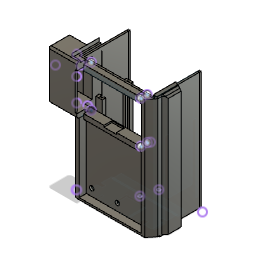
BAL-BOT-W-DISPLAY (Autodesk Fusion 360 design; units mm, degrees)
Autodesk Fusion 360 part; units mm, degrees
note: some values were not read from the file. Set by a fixed rule: which face or edge a step refers to.
(part 1 of 4)
sketch "Sketch1" plane through (0, 0, 0) normal (0, 1, 0) x (1, 0, 0)
  line L0 (0, 0) -> (-315, 0)
  line L1 (-315, 0) -> (-315, 66)
  line L2 (-315, 66) -> (0, 66)
  line L3 (0, 66) -> (0, 0)
  line L4 (-315, 0) -> (-272.5, 0)
  line L5 (-272.5, 0) -> (-272.5, -56.2)
  line L6 (-272.5, -56.2) -> (-315, -56.2)
  line L7 (-315, -56.2) -> (-315, 0)
  line L8 (0, 0) -> (-42.5, 0)
  line L9 (-42.5, 0) -> (-42.5, -56.2)
  line L10 (-42.5, -56.2) -> (0, -56.2)
  line L11 (0, -56.2) -> (0, 0)
  line L12 (-272.5, -56.2) -> (-42.5, -56.2)
  line L13 (-42.5, -56.2) -> (-42.5, 0)
  line L14 (-42.5, 0) -> (-272.5, 0)
  line L15 (-272.5, 0) -> (-272.5, -56.2)
  line L16 (-315, 0) -> (-272.5, -56.2)
  line L17 (0, 0) -> (-42.5, -56.2)
  dimension "d1" = 315
  dimension "d2" = 66
  dimension "d3" = 42.5
  dimension "d4" = 56.2
  dimension "d5" = 42.5
  dimension "d6" = 56.2
  constraint horizontal L0
  constraint vertical L1
  constraint horizontal L2
  constraint vertical L3
  constraint coincident L0.start L3.end
  constraint horizontal L4
  constraint vertical L5
  constraint horizontal L6
  constraint vertical L7
  constraint horizontal L8
  constraint vertical L9
  constraint horizontal L10
  constraint vertical L11
  constraint horizontal L12
  constraint vertical L13
  constraint horizontal L14
  constraint vertical L15
  measures "d1" distance of L0.start L0.end
  measures "d2" distance of L0.start L2.end
  measures "d3" distance of L0.end L4.end
  measures "d4" distance of L0.end L6.end
  measures "d5" distance of L0.start L8.end
  measures "d6" distance of L0.start L10.end
extrude "Extrude1" add sketch "Sketch1" along normal blind 5 contours L0 L8 L9 L13 L17 | L0 L1 L2 L3 L4 L8 L14 | L0 L5 L9 L12 L13 L14 L15 | L0 L4 L5 L15 L16 makes body 1
sketch "Sketch2" plane through (0, 5, 0) normal (0, 1, 0) x (-1, 0, 0)
  line L0 (315, 0) -> (272.5, 56.2)
  line L1 (272.5, 56.2) -> (42.5, 56.2)
  line L2 (42.5, 56.2) -> (0, 0)
  line L3 (0, 0) -> (0, -66)
  line L4 (0, -66) -> (315, -66)
  line L5 (315, -66) -> (315, 0)
  line L6 (272.5, 56.2) -> (272.5, -66)
  line L7 (42.5, 56.2) -> (42.5, -66)
  constraint coincident L0.end L1.start
  constraint coincident L4 L6.end
  constraint perpendicular L4 L6
  constraint coincident L1.end L2.start
  constraint coincident L4 L7.end
  constraint perpendicular L4 L7
extrude "Extrude2" cut sketch "Sketch2" against normal blind 5 contours L0 L4 L5 L6 | L2 L3 L4 L7 bodies 1
sketch "Sketch3" plane through (0, 5, 0) normal (0, 1, 0) x (-1, 0, 0)
  line L0 (272.5, -66) -> (272.5, 56.2)
  line L1 (272.5, 56.2) -> (42.5, 56.2)
  line L2 (42.5, 56.2) -> (42.5, -66)
  line L3 (42.5, -66) -> (272.5, -66)
  line L4 (42.5, -66) -> (152, -66)
  line L5 (152, -66) -> (152, -53.875)
  line L6 (152, -53.875) -> (42.5, -53.875)
  line L7 (42.5, -53.875) -> (42.5, -66)
  circle A0 centre (152, -53.875) radius 4
  line L8 (272.5, -66) -> (163, -66)
  line L9 (163, -66) -> (163, -12.125)
  line L10 (163, -12.125) -> (272.5, -12.125)
  line L11 (272.5, -12.125) -> (272.5, -66)
  circle A1 centre (163, -12.125) radius 4
  line L12 (272.5, -66) -> (259, -66)
  line L13 (259, -66) -> (259, -46)
  line L14 (259, -46) -> (272.5, -46)
  line L15 (272.5, -46) -> (272.5, -66)
  line L16 (259, -46) -> (56, -46)
  line L17 (56, -46) -> (56, -20)
  line L18 (56, -20) -> (259, -20)
  line L19 (259, -20) -> (259, -46)
  dimension "d11" = 109.5
  dimension "d12" = 12.125
  dimension "d13" = 8
  dimension "d14" = 109.5
  dimension "d15" = 53.875
  dimension "d16" = 8
  dimension "d17" = 13.5
  dimension "d18" = 20
  dimension "d19" = 203
  dimension "d20" = 26
  constraint horizontal L4
  constraint vertical L5
  constraint horizontal L6
  constraint vertical L7
  constraint coincident L2.end L3.start
  constraint coincident L5.end L6.start
  constraint horizontal L8
  constraint vertical L9
  constraint horizontal L10
  constraint vertical L11
  constraint coincident L0.start L3.end
  constraint coincident L9.end L10.start
  constraint horizontal L12
  constraint vertical L13
  constraint horizontal L14
  constraint vertical L15
  constraint horizontal L16
  constraint vertical L17
  constraint horizontal L18
  constraint vertical L19
  measures "d11" distance of L2.end L4.end
  measures "d12" distance of L2.end L6.end
  measures "d13" diameter of A0
  measures "d14" distance of L0.start L8.end
  measures "d15" distance of L0.start L10.end
  measures "d16" diameter of A1
  measures "d17" distance of L0.start L12.end
  measures "d18" distance of L0.start L14.end
  measures "d19" distance of L13.end L16.end
  measures "d20" distance of L13.end L18.end
extrude "Extrude3" cut sketch "Sketch3" against normal blind 5 contours L9 L16 L18 L19 | L9 L10 A1 | L9 L10 A1 | L9 L16 L17 L18 | L5 L6 A0 | L5 L6 A0 bodies 1
sketch "Sketch4" plane through (0, 0, 0) normal (0, -1, 0) x (1, 0, 0)
  line L0 (-56, -20) -> (-56, -46)
  line L1 (-56, -46) -> (-259, -46)
  line L2 (-259, -46) -> (-259, -20)
  line L3 (-259, -20) -> (-56, -20)
  circle A0 centre (-152, -53.875) radius 4
  circle A1 centre (-163, -12.125) radius 4
  line L4 (-272.5, 56.2) -> (-272.5, -66)
  line L5 (-272.5, -66) -> (-42.5, -66)
  line L6 (-42.5, -66) -> (-42.5, 56.2)
  line L7 (-42.5, 56.2) -> (-272.5, 56.2)
  line L8 (-42.5, 56.2) -> (-272.5, 56.2)
  line L9 (-272.5, 56.2) -> (-272.5, 51.2)
  line L10 (-272.5, 51.2) -> (-42.5, 51.2)
  line L11 (-42.5, 51.2) -> (-42.5, 56.2)
  line L12 (-42.5, 51.2) -> (-45, 51.2)
  line L13 (-45, 51.2) -> (-45, 3)
  line L14 (-45, 3) -> (-42.5, 3)
  line L15 (-42.5, 3) -> (-42.5, 51.2)
  line L16 (-272.5, 51.2) -> (-270, 51.2)
  line L17 (-270, 51.2) -> (-270, 3)
  line L18 (-270, 3) -> (-272.5, 3)
  line L19 (-272.5, 3) -> (-272.5, 51.2)
  line L20 (-45, 3) -> (-270, 3)
  line L21 (-270, 3) -> (-270, 51.2)
  line L22 (-270, 51.2) -> (-45, 51.2)
  line L23 (-45, 51.2) -> (-45, 3)
  dimension "d23" = 5
  dimension "d24" = 2.5
  dimension "d25" = 48.2
  dimension "d26" = 2.5
  dimension "d27" = 48.2
  constraint horizontal L8
  constraint vertical L9
  constraint horizontal L10
  constraint vertical L11
  constraint coincident L6.end L7.start
  constraint horizontal L12
  constraint vertical L13
  constraint horizontal L14
  constraint vertical L15
  constraint horizontal L16
  constraint vertical L17
  constraint horizontal L18
  constraint vertical L19
  constraint horizontal L20
  constraint vertical L21
  constraint horizontal L22
  constraint vertical L23
  measures "d23" distance of L6.end L10.end
  measures "d24" distance of L10.end L12.end
  measures "d25" distance of L10.end L14.end
  measures "d26" distance of L9.end L16.end
  measures "d27" distance of L9.end L18.end
extrude "Extrude4" cut sketch "Sketch4" against normal blind 5 contours L10 L13 L17 L20 L21 L22 L23 bodies 1
extrude "Extrude5" add 1 faces at (-270, 1.6667, 35.1333) along direction (1, 0, 0) blind 85 on bodies 1 bodies 1
extrude "Extrude6" add 1 faces at (-45, 1.6667, 35.1333) along direction (-1, 0, 0) blind 85 on bodies 1 bodies 1
sketch "Sketch5" plane through (0, 5, 0) normal (0, 1, 0) x (-1, 0, 0)
  line L0 (185, 3) -> (130, 3)
  line L1 (130, 3) -> (130, 51.2)
  line L2 (130, 51.2) -> (185, 51.2)
  line L3 (185, 51.2) -> (185, 3)
  line L4 (56, -46) -> (56, -20)
  line L5 (56, -20) -> (259, -20)
  line L6 (259, -20) -> (259, -46)
  line L7 (259, -46) -> (56, -46)
  circle A0 centre (152, -53.875) radius 4
  circle A1 centre (163, -12.125) radius 4
  line L8 (272.5, -66) -> (272.5, 56.2)
  line L9 (272.5, 56.2) -> (42.5, 56.2)
  line L10 (42.5, 56.2) -> (42.5, -66)
  line L11 (42.5, -66) -> (272.5, -66)
  line L12 (272.5, 56.2) -> (42.5, 56.2)
  line L13 (42.5, 56.2) -> (42.5, 51.2)
  line L14 (42.5, 51.2) -> (272.5, 51.2)
  line L15 (272.5, 51.2) -> (272.5, 56.2)
  dimension "d34" = 5
  constraint horizontal L12
  constraint vertical L13
  constraint horizontal L14
  constraint vertical L15
  constraint coincident L10 L13.end
  constraint coincident L8.end L9.start
  measures "d34" distance of L8.end L14.end
extrude "Extrude7" add sketch "Sketch5" along normal blind 150 contours L2 L8 L9 L10 L12 L13 L14 L15 bodies 1
sketch "Sketch6" plane through (0, 5, 0) normal (0, 1, 0) x (-1, 0, 0)
  line L0 (130, 51.2) -> (42.5, 51.2)
  line L1 (42.5, 51.2) -> (42.5, -66)
  line L2 (42.5, -66) -> (272.5, -66)
  line L3 (272.5, -66) -> (272.5, 51.2)
  line L4 (272.5, 51.2) -> (185, 51.2)
  line L5 (185, 51.2) -> (185, 3)
  line L6 (185, 3) -> (130, 3)
  line L7 (130, 3) -> (130, 51.2)
  line L8 (56, -46) -> (56, -20)
  line L9 (56, -20) -> (259, -20)
  line L10 (259, -20) -> (259, -46)
  line L11 (259, -46) -> (56, -46)
  circle A0 centre (152, -53.875) radius 4
  circle A1 centre (163, -12.125) radius 4
  line L12 (56, -20) -> (66, -20)
  line L13 (66, -20) -> (66, 51.2)
  line L14 (66, 51.2) -> (56, 51.2)
  line L15 (56, 51.2) -> (56, -20)
  line L16 (259, -20) -> (249, -20)
  line L17 (249, -20) -> (249, 51.2)
  line L18 (249, 51.2) -> (259, 51.2)
  line L19 (259, 51.2) -> (259, -20)
  point P0 (259, -20)
  dimension "d37" = 10
  dimension "d38" = 10
  dimension "d39" = 71.2
  constraint horizontal L12
  constraint vertical L13
  constraint horizontal L14
  constraint vertical L15
  constraint coincident L0 L13.end
  constraint coincident L8.end L9.start
  constraint horizontal L16
  constraint vertical L17
  constraint horizontal L18
  constraint vertical L19
  constraint coincident P0 L9.end
  measures "d37" distance of L8.end L12.end
  measures "d38" distance of P0 L16.end
  measures "d39" distance of P0 L18.end
extrude "Extrude8" add sketch "Sketch6" along normal blind 150 contours L0 L9 L12 L13 L14 L15 | L4 L9 L16 L17 L18 L19 bodies 1
sketch "Sketch7" plane through (-42.5, 0, 0) normal (1, 0, 0) x (0, 0, -1)
  line L0 (-56.2, 155) -> (-56.2, 0)
  line L1 (-56.2, 0) -> (66, 0)
  line L2 (66, 0) -> (66, 5)
  line L3 (66, 5) -> (-51.2, 5)
  line L4 (-51.2, 5) -> (-51.2, 155)
  line L5 (-51.2, 155) -> (-56.2, 155)
  line L6 (-51.2, 5) -> (-56.2, 5)
  line L7 (-56.2, 5) -> (-56.2, 155)
  line L8 (-56.2, 155) -> (-51.2, 155)
  line L9 (-51.2, 155) -> (-51.2, 5)
  constraint horizontal L6
  constraint vertical L7
  constraint horizontal L8
  constraint vertical L9
  constraint coincident L0.start L5.end
  constraint coincident L3.end L4.start
extrude "Extrude9" cut sketch "Sketch7" against normal blind 13.5 contours L0 L4 L5 L6 L7 L8 L9 bodies 1
sketch "Sketch8" plane through (-272.5, 0, 0) normal (-1, 0, 0) x (0, 0, 1)
  line L0 (51.2, 5) -> (-66, 5)
  line L1 (-66, 5) -> (-66, 0)
  line L2 (-66, 0) -> (56.2, 0)
  line L3 (56.2, 0) -> (56.2, 155)
  line L4 (56.2, 155) -> (51.2, 155)
  line L5 (51.2, 155) -> (51.2, 5)
  line L6 (51.2, 5) -> (56.2, 5)
  line L7 (56.2, 5) -> (56.2, 155)
  line L8 (56.2, 155) -> (51.2, 155)
  line L9 (51.2, 155) -> (51.2, 5)
  constraint horizontal L6
  constraint vertical L7
  constraint horizontal L8
  constraint vertical L9
  constraint coincident L3.end L4.start
  constraint coincident L0.start L5.end
extrude "Extrude10" cut sketch "Sketch8" against normal blind 13.5 contours L3 L4 L5 L6 L7 L8 L9 bodies 1
sketch "Sketch9" plane through (0, 0, -20) normal (0, 0, -1) x (-1, 0, 0)
  line L0 (56, 5) -> (56, 0)
  line L1 (56, 0) -> (259, 0)
  line L2 (259, 0) -> (259, 5)
  line L3 (259, 5) -> (259, 155)
  line L4 (259, 155) -> (249, 155)
  line L5 (249, 155) -> (249, 5)
  line L6 (249, 5) -> (66, 5)
  line L7 (66, 5) -> (66, 155)
  line L8 (66, 155) -> (56, 155)
  line L9 (56, 155) -> (56, 5)
  line L10 (56, 155) -> (66, 155)
  line L11 (66, 155) -> (66, 0)
  line L12 (66, 0) -> (56, 0)
  line L13 (56, 0) -> (56, 155)
  line L14 (249, 155) -> (259, 155)
  line L15 (259, 155) -> (259, 0)
  line L16 (259, 0) -> (249, 0)
  line L17 (249, 0) -> (249, 155)
  constraint horizontal L10
  constraint vertical L11
  constraint horizontal L12
  constraint vertical L13
  constraint coincident L1 L11.end
  constraint coincident L8.end L9.start
  constraint horizontal L14
  constraint vertical L15
  constraint horizontal L16
  constraint vertical L17
  constraint coincident L1.end L2.start
  constraint coincident L4.end L5.start
extrude "Extrude11" add sketch "Sketch9" along normal blind 25 contours L0 L1 L7 L8 L9 L10 L11 L12 L13 | L1 L2 L3 L4 L5 L14 L15 L16 L17 bodies 1
extrude "Extrude12" add 1 faces at (-62.6667, 53.3333, -45) along direction (0, 0, -1) blind 1 on bodies 1 bodies 1
extrude "Extrude13" add 1 faces at (-252.3333, 53.3333, -45) along direction (0, 0, -1) blind 1 on bodies 1 bodies 1
sketch "Sketch10" plane through (0, 0, 0) normal (0, -1, 0) x (1, 0, 0)
  line L0 (-185, 51.2) -> (-130, 51.2)
  line L1 (-130, 51.2) -> (-130, 3)
  line L2 (-130, 3) -> (-185, 3)
  line L3 (-185, 3) -> (-185, 51.2)
  line L4 (-66, -20) -> (-66, -46)
  line L5 (-66, -46) -> (-249, -46)
  line L6 (-249, -46) -> (-249, -20)
  line L7 (-249, -20) -> (-66, -20)
  circle A0 centre (-152, -53.875) radius 4
  circle A1 centre (-163, -12.125) radius 4
  line L8 (-42.5, -66) -> (-42.5, 56.2)
  line L9 (-42.5, 56.2) -> (-272.5, 56.2)
extrude "Extrude14" add 1 faces at (-62.6667, 105, -46) along direction (0, 0, -1) blind 20 on bodies 1 bodies 1
extrude "Extrude15" add 1 faces at (-252.3333, 55, -46) along direction (0, 0, -1) blind 20 on bodies 1 bodies 1
sketch "Sketch11" plane through (0, 5, 0) normal (0, 1, 0) x (-1, 0, 0)
  line L0 (249, -66) -> (249, -46)
  line L1 (249, -46) -> (66, -46)
  line L2 (66, -46) -> (66, -66)
  line L3 (66, -66) -> (249, -66)
  circle A0 centre (152, -53.875) radius 4
  line L4 (66, -66) -> (249, -66)
  line L5 (249, -66) -> (249, -61)
  line L6 (249, -61) -> (66, -61)
  line L7 (66, -61) -> (66, -66)
  dimension "d56" = 5
  constraint horizontal L4
  constraint vertical L5
  constraint horizontal L6
  constraint vertical L7
  constraint coincident L2.end L3.start
  measures "d56" distance of L2.end L6.end
extrude "Extrude16" add sketch "Sketch11" along normal blind 30 contours L0 L2 L3 L4 L5 L6 L7 bodies 1
sketch "Sketch12" plane through (0, 0, -66) normal (0, 0, -1) x (-1, 0, 0)
  line L0 (272.5, 0) -> (272.5, 5)
  line L1 (272.5, 5) -> (259, 5)
  line L2 (259, 5) -> (259, 155)
  line L3 (259, 155) -> (249, 155)
  line L4 (249, 155) -> (249, 35)
  line L5 (249, 35) -> (66, 35)
  line L6 (66, 35) -> (66, 155)
  line L7 (66, 155) -> (56, 155)
  line L8 (56, 155) -> (56, 5)
  line L9 (56, 5) -> (42.5, 5)
  line L10 (42.5, 5) -> (42.5, 0)
  line L11 (42.5, 0) -> (272.5, 0)
  line L12 (66, 5, -117.2) -> (157.5, 5, -117.2)
  line L13 (157.5, 5, -117.2) -> (157.5, 25, -117.2)
  line L14 (157.5, 25, -117.2) -> (66, 25, -117.2)
  line L15 (66, 25, -117.2) -> (66, 5, -117.2)
  circle A0 through (163, 25, -117.2) (154.75, 29.7631, -117.2) (154.75, 20.2369, -117.2)
  point P0 (66, 5)
  dimension "d59" = 20
  dimension "d60" = 11
extrude "Extrude17" cut sketch "Sketch12" against normal blind 5 contours L13 L14 A0 | L13 L14 A0 in plane through (0, 0, 51.2) normal (0, 0, -1) bodies 1
sketch "Sketch13" plane through (0, 0, 0) normal (0, -1, 0) x (1, 0, 0)
  line L0 (-130, 3) -> (-45, 3)
  line L1 (-45, 3) -> (-45, 51.2)
  line L2 (-45, 51.2) -> (-130, 51.2)
  line L3 (-130, 51.2) -> (-130, 3)
  line L4 (-185, 3) -> (-270, 3)
  line L5 (-270, 3) -> (-270, 51.2)
  line L6 (-270, 51.2) -> (-185, 51.2)
  line L7 (-185, 51.2) -> (-185, 3)
  point P0 (-130, 3)
  point P1 (-185, 3)
  dimension "d63" = 85
  dimension "d64" = 85
  constraint horizontal L0
  constraint vertical L1
  constraint horizontal L2
  constraint vertical L3
  constraint coincident P0 L0.start
  constraint horizontal L4
  constraint vertical L5
  constraint horizontal L6
  constraint vertical L7
  constraint coincident P1 L4.start
  measures "d63" distance of P0 L0.end
  measures "d64" distance of P1 L4.end
extrude "Extrude18" add sketch "Sketch13" along normal blind 3 bodies 1
sketch "Sketch14" plane through (0, 0, 51.2) normal (0, 0, -1) x (-1, 0, 0)
  circle A0 centre (157.5, 25) radius 5.5
  line L0 (249, 5) -> (249, 155)
  line L1 (249, 155) -> (66, 155)
  line L2 (66, 155) -> (66, 5)
  line L3 (66, 5) -> (130, 5)
  line L4 (130, 5) -> (130, 0)
  line L5 (130, 0) -> (185, 0)
  line L6 (185, 0) -> (185, 5)
  line L7 (185, 5) -> (249, 5)
  line L8 (249, 155) -> (218, 155)
  line L9 (218, 155) -> (218, 5)
  line L10 (218, 5) -> (249, 5)
  line L11 (249, 5) -> (249, 155)
  line L12 (66, 155) -> (97, 155)
  line L13 (97, 155) -> (97, 5)
  line L14 (97, 5) -> (66, 5)
  line L15 (66, 5) -> (66, 155)
  line L16 (218, 155) -> (97, 155)
  line L17 (97, 155) -> (97, 65.5)
  line L18 (97, 65.5) -> (218, 65.5)
  line L19 (218, 65.5) -> (218, 155)
  line L20 (218, 65.5) -> (223, 65.5)
  line L21 (223, 65.5) -> (223, 155)
  line L22 (223, 155) -> (218, 155)
  line L23 (218, 155) -> (218, 65.5)
  line L24 (97, 65.5) -> (92, 65.5)
  line L25 (92, 65.5) -> (92, 155)
  line L26 (92, 155) -> (97, 155)
  line L27 (97, 155) -> (97, 65.5)
  line L28 (92, 65.5) -> (223, 65.5)
  line L29 (223, 65.5) -> (223, 60.5)
  line L30 (223, 60.5) -> (92, 60.5)
  line L31 (92, 60.5) -> (92, 65.5)
  dimension "d67" = 31
  dimension "d68" = 31
  dimension "d69" = 89.5
  dimension "d70" = 5
  dimension "d71" = 5
  dimension "d72" = 5
  constraint horizontal L8
  constraint vertical L9
  constraint horizontal L10
  constraint vertical L11
  constraint coincident L0.end L1.start
  constraint horizontal L12
  constraint vertical L13
  constraint horizontal L14
  constraint vertical L15
  constraint coincident L1.end L2.start
  constraint horizontal L16
  constraint vertical L17
  constraint horizontal L18
  constraint vertical L19
  constraint horizontal L20
  constraint vertical L21
  constraint horizontal L22
  constraint vertical L23
  constraint horizontal L24
  constraint vertical L25
  constraint horizontal L26
  constraint vertical L27
  constraint horizontal L28
  constraint vertical L29
  constraint horizontal L30
  constraint vertical L31
  measures "d67" distance of L0.end L8.end
  measures "d68" distance of L1.end L12.end
  measures "d69" distance of L8.end L18.end
  measures "d70" distance of L18.end L20.end
  measures "d71" distance of L17.end L24.end
  measures "d72" distance of L24.end L30.end
extrude "Extrude19" add sketch "Sketch14" along normal blind 10 contours L1 L8 L9 L19 L20 L21 L22 L23 L28 | L9 L13 L18 L28 L30 | L9 L20 L28 L29 L30 | L13 L24 L28 L30 L31 | L1 L12 L13 L17 L24 L25 L26 L27 L28 bodies 1
extrude "Extrude20" add 1 faces at (-137.3333, 62.1667, 41.2) along direction (0, 0, -1) blind 3 on bodies 1 bodies 1
sketch "Sketch15" plane through (0, 0, 38.2) normal (0, 0, -1) x (-1, 0, 0)
  line L0 (223, 60.5) -> (223, 155)
  line L1 (223, 155) -> (218, 155)
  line L2 (218, 155) -> (218, 65.5)
  line L3 (218, 65.5) -> (97, 65.5)
  line L4 (97, 65.5) -> (97, 155)
  line L5 (97, 155) -> (92, 155)
  line L6 (92, 155) -> (92, 60.5)
  line L7 (92, 60.5) -> (223, 60.5)
  line L8 (223, 60.5) -> (213, 60.5)
  line L9 (213, 60.5) -> (213, 155)
  line L10 (213, 155) -> (223, 155)
  line L11 (223, 155) -> (223, 60.5)
  line L12 (92, 60.5) -> (102, 60.5)
  line L13 (102, 60.5) -> (102, 155)
  line L14 (102, 155) -> (92, 155)
  line L15 (92, 155) -> (92, 60.5)
  dimension "d77" = 10
  dimension "d78" = 10
  constraint horizontal L8
  constraint vertical L9
  constraint horizontal L10
  constraint vertical L11
  constraint coincident L0.start L7.end
  constraint horizontal L12
  constraint vertical L13
  constraint horizontal L14
  constraint vertical L15
  constraint coincident L6.end L7.start
  measures "d77" distance of L0.start L8.end
  measures "d78" distance of L6.end L12.end
extrude "Extrude21" add sketch "Sketch15" along normal blind 5.9 contours L0 L1 L2 L3 L7 L8 L9 L10 L11 | L2 L3 L9 L10 | L3 L4 L5 L6 L7 L12 L13 L14 L15 | L3 L4 L13 L14 bodies 1
sketch "Sketch16" plane through (-42.5, 0, 0) normal (1, 0, 0) x (0, 0, -1)
  line L0 (66, 5) -> (-56.2, 5)
  line L1 (-56.2, 5) -> (-56.2, 0)
  line L2 (-56.2, 0) -> (66, 0)
  line L3 (66, 0) -> (66, 5)
  line L4 (66, 5) -> (-3, 5)
  line L5 (-3, 5) -> (-3, 0)
  line L6 (-3, 0) -> (66, 0)
  line L7 (66, 0) -> (66, 5)
  dimension "d81" = 69
  constraint horizontal L4
  constraint vertical L5
  constraint horizontal L6
  constraint vertical L7
  constraint coincident L0.start L3.end
  measures "d81" distance of L0.start L4.end
extrude "Extrude22" cut sketch "Sketch16" against normal blind 13 contours L0 L2 L3 L4 L5 L6 L7 bodies 1
sketch "Sketch17" plane through (-157.5, 0, -33) normal (0, -1, 0) x (1, 0, 0)
  line L0 (-115, -33) -> (-115, 36)
  line L1 (-115, 36, 0) -> (-115, 36, -5)
  line L2 (-115, 36, -5) -> (-115, -33, -5)
  line L3 (-115, -33, -5) -> (-115, -33, 0)
  point P0 (-115, -33)
  dimension "d84" = 69
  constraint vertical L0
  constraint coincident P0 L0.start
  measures "d84" distance of P0 L0.end
extrude "Extrude23" cut sketch "Sketch17" along normal blind 13 contours L0 L1 L2 L3 in plane through (-272.5, 0, -33) normal (1, 0, 0) bodies 1
extrude "Extrude24" cut 1 faces at (-259.5, 1.6667, -43) along direction (1, 0, 0) blind 0.5 on bodies 1 bodies 1
extrude "Extrude25" cut 1 faces at (-55.5, 3.3333, -20) along direction (-1, 0, 0) blind 0.5 on bodies 1 bodies 1
sketch "Sketch18" plane through (0, 0, 56.2) normal (0, 0, 1) x (1, 0, 0)
  circle A0 centre (-157.5, 25) radius 5.5
  line L0 (-259, 5) -> (-272.5, 5)
  line L1 (-272.5, 5) -> (-272.5, 0)
  line L2 (-272.5, 0) -> (-42.5, 0)
  line L3 (-42.5, 0) -> (-42.5, 5)
  line L4 (-42.5, 5) -> (-56, 5)
  line L5 (-56, 5) -> (-56, 155)
  line L6 (-56, 155) -> (-259, 155)
  line L7 (-259, 155) -> (-259, 5)
  line L8 (-249, 5, -5) -> (-229, 5, -5)
  line L9 (-229, 5, -5) -> (-229, 25, -5)
  line L10 (-229, 25, -5) -> (-249, 25, -5)
  line L11 (-249, 25, -5) -> (-249, 5, -5)
  circle A1 through (-223.35, 25, -5) (-231.825, 29.893, -5) (-231.825, 20.107, -5)
  point P0 (-249, 5)
  dimension "d91" = 20
  dimension "d92" = 20
  dimension "d93" = 11.3
extrude "Extrude26" cut sketch "Sketch18" along normal blind 5 contours L9 L10 A1 | L9 L10 A1 in plane through (0, 0, 51.2) normal (0, 0, 1) bodies 1
sketch "Sketch19" plane through (-249, 0, 0) normal (1, 0, 0) x (0, 0, -1)
  line L0 (61, 35) -> (66, 35)
  line L1 (66, 35) -> (66, 155)
  line L2 (66, 155) -> (-51.2, 155)
  line L3 (-51.2, 155) -> (-51.2, 5)
  line L4 (-51.2, 5) -> (20, 5)
  line L5 (20, 5) -> (20, 0)
  line L6 (20, 0) -> (46, 0)
  line L7 (46, 0) -> (46, 5)
  line L8 (46, 5) -> (61, 5)
  line L9 (61, 5) -> (61, 35)
  line L10 (-51.2, 155) -> (-30, 155)
  line L11 (-30, 155) -> (-30, 5)
  line L12 (-30, 5) -> (-51.2, 5)
  line L13 (-51.2, 5) -> (-51.2, 155)
  line L14 (-30, 155) -> (46, 155)
  line L15 (46, 155) -> (46, 83)
  line L16 (46, 83) -> (-30, 83)
  line L17 (-30, 83) -> (-30, 155)
  line L18 (-30, 155) -> (-35, 155)
  line L19 (-35, 155) -> (-35, 78)
  line L20 (-35, 78) -> (-30, 78)
  line L21 (-30, 78) -> (-30, 155)
  line L22 (46, 155) -> (51, 155)
  line L23 (51, 155) -> (51, 78)
  line L24 (51, 78) -> (46, 78)
  line L25 (46, 78) -> (46, 155)
  line L26 (-30, 83) -> (46, 83)
  line L27 (46, 83) -> (46, 78)
  line L28 (46, 78) -> (-30, 78)
  line L29 (-30, 78) -> (-30, 83)
  dimension "d96" = 21.2
  dimension "d97" = 76
  dimension "d98" = 72
  dimension "d99" = 5
  dimension "d100" = 77
  dimension "d101" = 5
  dimension "d102" = 77
  constraint horizontal L10
  constraint vertical L11
  constraint horizontal L12
  constraint vertical L13
  constraint coincident L2.end L3.start
  constraint horizontal L14
  constraint vertical L15
  constraint horizontal L16
  constraint vertical L17
  constraint horizontal L18
  constraint vertical L19
  constraint horizontal L20
  constraint vertical L21
  constraint horizontal L22
  constraint vertical L23
  constraint horizontal L24
  constraint vertical L25
  constraint horizontal L26
  constraint vertical L27
  constraint horizontal L28
  constraint vertical L29
  measures "d96" distance of L2.end L10.end
  measures "d97" distance of L10.end L14.end
  measures "d98" distance of L10.end L16.end
  measures "d99" distance of L10.end L18.end
  measures "d100" distance of L10.end L20.end
  measures "d101" distance of L14.end L22.end
  measures "d102" distance of L14.end L24.end
extrude "Extrude27" add sketch "Sketch19" along normal blind 5 contours L2 L15 L22 L23 L24 L25 L27 | L2 L10 L11 L17 L18 L19 L20 L21 L29 | L11 L16 L21 L25 L26 L27 L28 L29 bodies 1
extrude "Extrude28" cut 1 faces at (-249, 131, -20.6667) along direction (-1, 0, 0) blind 5 on bodies 1 bodies 1
sketch "Sketch20" plane through (-254, 0, 0) normal (1, 0, 0) x (0, 0, -1)
  line L0 (46, 83) -> (46, 155)
  line L1 (46, 155) -> (-30, 155)
  line L2 (-30, 155) -> (-30, 83)
  line L3 (-30, 83) -> (46, 83)
  line L4 (-30, 155) -> (-25, 155)
  line L5 (-25, 155) -> (-25, 83)
  line L6 (-25, 83) -> (-30, 83)
  line L7 (-30, 83) -> (-30, 155)
  line L8 (46, 155) -> (41, 155)
  line L9 (41, 155) -> (41, 83)
  line L10 (41, 83) -> (46, 83)
  line L11 (46, 83) -> (46, 155)
  dimension "d107" = 5
  dimension "d108" = 5
  constraint horizontal L4
  constraint vertical L5
  constraint horizontal L6
  constraint vertical L7
  constraint coincident L1.end L2.start
  constraint horizontal L8
  constraint vertical L9
  constraint horizontal L10
  constraint vertical L11
  constraint coincident L0.end L1.start
  measures "d107" distance of L1.end L4.end
  measures "d108" distance of L0.end L8.end
extrude "Extrude29" add sketch "Sketch20" along normal blind 5 contours L0 L1 L3 L8 L9 L10 L11 | L1 L2 L3 L4 L5 L6 L7 bodies 1
extrude "Extrude30" add 1 faces at (-244, 79.6667, 4.6667) along direction (1, 0, 0) blind 5 on bodies 1 bodies 1
extrude "Extrude31" add 1 faces at (-249, 107, 28.3333) along direction (1, 0, 0) blind 3 on bodies 1 bodies 1
extrude "Extrude32" add 1 faces at (-249, 107, -42.6667) along direction (1, 0, 0) blind 3 on bodies 1 bodies 1
extrude "Extrude33" add 1 faces at (-239, 79.6667, 4.6667) along direction (1, 0, 0) blind 3 on bodies 1 bodies 1
sketch "Sketch21" plane through (0, 0, 30) normal (0, 0, -1) x (-1, 0, 0)
  line L0 (246, 83) -> (246, 155)
  line L1 (246, 155) -> (236, 155)
  line L2 (236, 155) -> (236, 83)
  line L3 (236, 83) -> (246, 83)
  line L4 (236, 83) -> (241, 83)
  line L5 (241, 83) -> (241, 155)
  line L6 (241, 155) -> (236, 155)
  line L7 (236, 155) -> (236, 83)
  constraint horizontal L4
  constraint vertical L5
  constraint horizontal L6
  constraint vertical L7
  constraint midpoint L1 L5.end
  constraint coincident L2.end L3.start
extrude "Extrude34" add sketch "Sketch21" along normal blind 5 contours L1 L2 L3 L4 L5 L6 L7 bodies 1
sketch "Sketch22" plane through (0, 0, -46) normal (0, 0, 1) x (1, 0, 0)
  line L0 (-246, 155) -> (-246, 83)
  line L1 (-246, 83) -> (-236, 83)
  line L2 (-236, 83) -> (-236, 155)
  line L3 (-236, 155) -> (-246, 155)
  line L4 (-236, 83) -> (-241, 83)
  line L5 (-241, 83) -> (-241, 155)
  line L6 (-241, 155) -> (-236, 155)
  line L7 (-236, 155) -> (-236, 83)
  constraint horizontal L4
  constraint vertical L5
  constraint horizontal L6
  constraint vertical L7
  constraint midpoint L3 L5.end
  constraint coincident L1.end L2.start
extrude "Extrude35" add sketch "Sketch22" along normal blind 5 contours L1 L2 L3 L4 L5 L6 L7 bodies 1
extrude "Extrude36" cut 1 faces at (-246, 107, -42.6667) along direction (-1, 0, 0) blind 0.2 on bodies 1 bodies 1
extrude "Extrude37" cut 1 faces at (-246, 107, 28.3333) along direction (-1, 0, 0) blind 0.2 on bodies 1 bodies 1
sketch "Sketch23" plane through (-236, 0, 0) normal (1, 0, 0) x (0, 0, -1)
  line L0 (-25, 155) -> (-35, 155)
  line L1 (-35, 155) -> (-35, 78)
  line L2 (-35, 78) -> (51, 78)
  line L3 (51, 78) -> (51, 155)
  line L4 (51, 155) -> (41, 155)
  line L5 (41, 155) -> (41, 83)
  line L6 (41, 83) -> (-25, 83)
  line L7 (-25, 83) -> (-25, 155)
  line L8 (-25, 83) -> (41, 83)
  line L9 (41, 83) -> (41, 78)
  line L10 (41, 78) -> (-25, 78)
  line L11 (-25, 78) -> (-25, 83)
  constraint horizontal L8
  constraint vertical L9
  constraint horizontal L10
  constraint vertical L11
  constraint coincident L2 L9.end
  constraint coincident L6.end L7.start
extrude "Extrude38" cut sketch "Sketch23" against normal blind 15 contours L2 L6 L8 L9 L10 L11 bodies 1
sketch "Sketch24" plane through (-66, 0, 0) normal (-1, 0, 0) x (0, 0, 1)
  line L0 (-66, 35) -> (-61, 35)
  line L1 (-61, 35) -> (-61, 5)
  line L2 (-61, 5) -> (-46, 5)
  line L3 (-46, 5) -> (-46, 0)
  line L4 (-46, 0) -> (-20, 0)
  line L5 (-20, 0) -> (-20, 5)
  line L6 (-20, 5) -> (51.2, 5)
  line L7 (51.2, 5) -> (51.2, 155)
  line L8 (51.2, 155) -> (-66, 155)
  line L9 (-66, 155) -> (-66, 35)
  line L10 (-66, 35) -> (-41, 35)
  line L11 (-41, 35) -> (-41, 155)
  line L12 (-41, 155) -> (-66, 155)
  line L13 (-66, 155) -> (-66, 35)
  line L14 (-66, 155) -> (-51, 155)
  line L15 (-51, 155) -> (-51, 35)
  line L16 (-51, 35) -> (-66, 35)
  line L17 (-66, 35) -> (-66, 155)
  dimension "d129" = 25
  dimension "d130" = 15
  constraint horizontal L10
  constraint vertical L11
  constraint horizontal L12
  constraint vertical L13
  constraint coincident L0.start L9.end
  constraint horizontal L14
  constraint vertical L15
  constraint horizontal L16
  constraint vertical L17
  measures "d129" distance of L0.start L10.end
  measures "d130" distance of L8.end L14.end
extrude "Extrude39" add sketch "Sketch24" along normal blind 13 contours L8 L10 L11 L12 L15 bodies 1
sketch "Sketch25" plane through (-66, 0, 0) normal (-1, 0, 0) x (0, 0, 1)
  line L0 (-41, 155) -> (-41, 35)
  line L1 (-41, 35) -> (-51, 35)
  line L2 (-51, 35) -> (-51, 155)
  line L3 (-51, 155) -> (-66, 155)
  line L4 (-66, 155) -> (-66, 35)
  line L5 (-66, 35) -> (-61, 35)
  line L6 (-61, 35) -> (-61, 5)
  line L7 (-61, 5) -> (-46, 5)
  line L8 (-46, 5) -> (-46, 0)
  line L9 (-46, 0) -> (-20, 0)
  line L10 (-20, 0) -> (-20, 5)
  line L11 (-20, 5) -> (51.2, 5)
  line L12 (51.2, 5) -> (51.2, 155)
  line L13 (51.2, 155) -> (-41, 155)
  line L14 (-41, 155) -> (25, 155)
  line L15 (25, 155) -> (25, 35)
  line L16 (25, 35) -> (-41, 35)
  line L17 (-41, 35) -> (-41, 155)
  line L18 (25, 155) -> (35, 155)
  line L19 (35, 155) -> (35, 35)
  line L20 (35, 35) -> (25, 35)
  line L21 (25, 35) -> (25, 155)
  dimension "d133" = 66
  dimension "d134" = 10
  constraint horizontal L14
  constraint vertical L15
  constraint horizontal L16
  constraint vertical L17
  constraint coincident L0.start L13.end
  constraint horizontal L18
  constraint vertical L19
  constraint horizontal L20
  constraint vertical L21
  measures "d133" distance of L0.start L14.end
  measures "d134" distance of L14.end L18.end
extrude "Extrude40" add sketch "Sketch25" along normal blind 13 contours L13 L15 L18 L19 L20 L21 bodies 1
extrude "Extrude41" cut 1 faces at (-251, 79.6667, -19) along direction (-1, 0, 0) blind 2.5 on bodies 1 bodies 1
extrude "Extrude42" cut 1 faces at (-253.5, 79.6667, -19) along direction (-1, 0, 0) blind 0.5 on bodies 1 bodies 1
sketch "Sketch26" plane through (-66, 0, 0) normal (-1, 0, 0) x (0, 0, 1)
  line L0 (35, 155) -> (35, 35)
  line L1 (35, 35) -> (25, 35)
  line L2 (25, 35) -> (25, 155)
  line L3 (25, 155) -> (-41, 155)
  line L4 (-41, 155) -> (-41, 35)
  line L5 (-41, 35) -> (-51, 35)
  line L6 (-51, 35) -> (-51, 155)
  line L7 (-51, 155) -> (-66, 155)
  line L8 (-66, 155) -> (-66, 35)
  line L9 (-66, 35) -> (-61, 35)
  line L10 (-61, 35) -> (-61, 5)
  line L11 (-61, 5) -> (-46, 5)
  line L12 (-46, 5) -> (-46, 0)
  line L13 (-46, 0) -> (-20, 0)
  line L14 (-20, 0) -> (-20, 5)
  line L15 (-20, 5) -> (51.2, 5)
  line L16 (51.2, 5) -> (51.2, 155)
  line L17 (51.2, 155) -> (35, 155)
  line L18 (25, 155) -> (-41, 155)
  line L19 (-41, 155) -> (-41, 78)
  line L20 (-41, 78) -> (25, 78)
  line L21 (25, 78) -> (25, 155)
  dimension "d141" = 77
  constraint horizontal L18
  constraint vertical L19
  constraint horizontal L20
  constraint vertical L21
  constraint coincident L2.end L3.start
  measures "d141" distance of L2.end L20.end
extrude "Extrude43" cut sketch "Sketch26" against normal blind 5 contours L2 L3 L4 L18 L19 L20 L21 bodies 1
sketch "Sketch27" plane through (0, 155, 0) normal (0, 1, 0) x (-1, 0, 0)
  line L0 (61, 25) -> (79, 25)
  line L1 (79, 25) -> (79, 35)
  line L2 (79, 35) -> (66, 35)
  line L3 (66, 35) -> (66, 51.2)
  line L4 (66, 51.2) -> (92, 51.2)
  line L5 (92, 51.2) -> (92, 32.3)
  line L6 (92, 32.3) -> (102, 32.3)
  line L7 (102, 32.3) -> (102, 38.2)
  line L8 (102, 38.2) -> (97, 38.2)
  line L9 (97, 38.2) -> (97, 51.2)
  line L10 (97, 51.2) -> (218, 51.2)
  line L11 (218, 51.2) -> (218, 38.2)
  line L12 (218, 38.2) -> (213, 38.2)
  line L13 (213, 38.2) -> (213, 32.3)
  line L14 (213, 32.3) -> (223, 32.3)
  line L15 (223, 32.3) -> (223, 51.2)
  line L16 (223, 51.2) -> (249, 51.2)
  line L17 (249, 51.2) -> (249, 35)
  line L18 (249, 35) -> (236, 35)
  line L19 (236, 35) -> (236, 25)
  line L20 (236, 25) -> (241, 25)
  line L21 (241, 25) -> (241, 30)
  line L22 (241, 30) -> (246.2, 30)
  line L23 (246.2, 30) -> (246.2, 25)
  line L24 (246.2, 25) -> (254, 25)
  line L25 (254, 25) -> (254, -41)
  line L26 (254, -41) -> (246.2, -41)
  line L27 (246.2, -41) -> (246.2, -46)
  line L28 (246.2, -46) -> (241, -46)
  line L29 (241, -46) -> (241, -41)
  line L30 (241, -41) -> (236, -41)
  line L31 (236, -41) -> (236, -51)
  line L32 (236, -51) -> (249, -51)
  line L33 (249, -51) -> (249, -66)
  line L34 (249, -66) -> (259, -66)
  line L35 (259, -66) -> (259, 56.2)
  line L36 (259, 56.2) -> (56, 56.2)
  line L37 (56, 56.2) -> (56, -66)
  line L38 (56, -66) -> (66, -66)
  line L39 (66, -66) -> (66, -51)
  line L40 (66, -51) -> (79, -51)
  line L41 (79, -51) -> (79, -41)
  line L42 (79, -41) -> (61, -41)
  line L43 (61, -41) -> (61, 25)
  line L44 (79, -41) -> (74, -41)
  line L45 (74, -41) -> (74, -51)
  line L46 (74, -51) -> (79, -51)
  line L47 (79, -51) -> (79, -41)
  line L48 (79, -41) -> (56, -41)
  line L49 (56, -41) -> (56, -46)
  line L50 (56, -46) -> (79, -46)
  line L51 (79, -46) -> (79, -41)
  line L52 (74, -46) -> (68.8, -46)
  line L53 (68.8, -46) -> (68.8, -41)
  line L54 (68.8, -41) -> (74, -41)
  line L55 (74, -41) -> (74, -46)
  line L56 (79, 25) -> (56, 25)
  line L57 (56, 25) -> (56, 30)
  line L58 (56, 30) -> (79, 30)
  line L59 (79, 30) -> (79, 25)
  line L60 (79, 35) -> (74, 35)
  line L61 (74, 35) -> (74, 25)
  line L62 (74, 25) -> (79, 25)
  line L63 (79, 25) -> (79, 35)
  line L64 (74, 25) -> (68.8, 25)
  line L65 (68.8, 25) -> (68.8, 30)
  line L66 (68.8, 30) -> (74, 30)
  line L67 (74, 30) -> (74, 25)
  dimension "d144" = 5
  dimension "d145" = 5
  dimension "d146" = 5.2
  dimension "d147" = 5
  dimension "d148" = 5
  dimension "d149" = 5.2
  constraint horizontal L44
  constraint vertical L45
  constraint horizontal L46
  constraint vertical L47
  constraint coincident L41.end L42.start
  constraint horizontal L48
  constraint vertical L49
  constraint horizontal L50
  constraint vertical L51
  constraint horizontal L52
  constraint vertical L53
  constraint horizontal L54
  constraint vertical L55
  constraint midpoint L45 L52.start
  constraint horizontal L56
  constraint vertical L57
  constraint horizontal L58
  constraint vertical L59
  constraint coincident L0.end L1.start
  constraint horizontal L60
  constraint vertical L61
  constraint horizontal L62
  constraint vertical L63
  constraint coincident L1.end L2.start
  constraint horizontal L64
  constraint vertical L65
  constraint horizontal L66
  constraint vertical L67
  measures "d144" distance of L41.end L44.end
  measures "d145" distance of L41.end L50.end
  measures "d146" distance of L52.start L52.end
  measures "d147" distance of L0.end L58.end
  measures "d148" distance of L1.end L60.end
  measures "d149" distance of L61.end L64.end
extrude "Extrude44" cut sketch "Sketch27" against normal blind 72 contours L0 L56 L58 L61 L64 L65 L66 L67 | L42 L45 L48 L50 L52 L53 L54 L55 bodies 1
sketch "Sketch28" plane through (0, 0, 25) normal (0, 0, -1) x (-1, 0, 0)
  line L0 (74, 155) -> (74, 83)
  line L1 (74, 83) -> (68.8, 83)
  line L2 (68.8, 83) -> (68.8, 155)
  line L3 (68.8, 155) -> (61, 155)
  line L4 (61, 155) -> (61, 78)
  line L5 (61, 78) -> (66, 78)
  line L6 (66, 78) -> (66, 35)
  line L7 (66, 35) -> (79, 35)
  line L8 (79, 35) -> (79, 155)
  line L9 (79, 155) -> (74, 155)
  line L10 (66, 78) -> (79, 78)
  line L11 (79, 78) -> (79, 35)
  line L12 (79, 35) -> (66, 35)
  line L13 (66, 35) -> (66, 78)
  constraint horizontal L10
  constraint vertical L11
  constraint horizontal L12
  constraint vertical L13
  constraint coincident L7.end L8.start
  constraint coincident L5.end L6.start
extrude "Extrude45" cut sketch "Sketch28" against normal blind 10 contours L6 L7 L8 L10 L11 L12 L13 bodies 1
sketch "Sketch29" plane through (0, 0, -41) normal (0, 0, 1) x (1, 0, 0)
  line L0 (-68.8, 155) -> (-68.8, 83)
  line L1 (-68.8, 83) -> (-74, 83)
  line L2 (-74, 83) -> (-74, 155)
  line L3 (-74, 155) -> (-79, 155)
  line L4 (-79, 155) -> (-79, 35)
  line L5 (-79, 35) -> (-66, 35)
  line L6 (-66, 35) -> (-66, 78)
  line L7 (-66, 78) -> (-61, 78)
  line L8 (-61, 78) -> (-61, 155)
  line L9 (-61, 155) -> (-68.8, 155)
  line L10 (-79, 35) -> (-66, 35)
  line L11 (-66, 35) -> (-66, 78)
  line L12 (-66, 78) -> (-79, 78)
  line L13 (-79, 78) -> (-79, 35)
  constraint horizontal L10
  constraint vertical L11
  constraint horizontal L12
  constraint vertical L13
  constraint coincident L6.end L7.start
  constraint coincident L4.end L5.start
extrude "Extrude46" cut sketch "Sketch29" against normal blind 10 contours L4 L5 L6 L10 L11 L12 L13 bodies 1
extrude "Extrude47" add 1 faces at (-70.3333, 129.3333, -51) along direction (0, 0, -1) blind 5 on bodies 1 bodies 1
extrude "Extrude48" add 1 faces at (-240.3333, 103.6667, -51) along direction (0, 0, -1) blind 5 on bodies 1 bodies 1
extrude "Extrude49" add 1 faces at (-244.6667, 78, 28.3333) along direction (0, -1, 0) blind 8 on bodies 1 bodies 1
extrude "Extrude50" add 1 faces at (-240.3333, 78, -46) along direction (0, -1, 0) blind 8 on bodies 1 bodies 1
extrude "Extrude51" cut 1 faces at (-250.6667, 78, 3) along direction (0, -1, 0) blind 8 on bodies 1 bodies 1
extrude "Extrude52" cut 1 faces at (-244.4667, 83, 26.6667) along direction (0, -1, 0) blind 8 on bodies 1 bodies 1
extrude "Extrude53" add 1 faces at (-244.6667, 70, 28.3333) along direction (0, -1, 0) blind 8 on bodies 1 bodies 1
extrude "Extrude54" add 1 faces at (-240.3333, 70, -46) along direction (0, -1, 0) blind 8 on bodies 1 bodies 1
extrude "Extrude55" cut 1 faces at (-250.6667, 70, 3) along direction (0, -1, 0) blind 8 on bodies 1 bodies 1
extrude "Extrude56" cut 1 faces at (-244.4667, 75, 26.6667) along direction (0, -1, 0) blind 8 on bodies 1 bodies 1
extrude "Extrude57" cut 1 faces at (-244.4667, 83, -44.3333) along direction (0, -1, 0) blind 8 on bodies 1 bodies 1
extrude "Extrude58" cut 1 faces at (-246.2, 96.3333, 28.3333) along direction (-1, 0, 0) blind 0.8 on bodies 1 bodies 1
extrude "Extrude59" cut 1 faces at (-246.2, 128.3333, -42.6667) along direction (-1, 0, 0) blind 0.8 on bodies 1 bodies 1
extrude "Extrude60" add 1 faces at (-74.6667, 78, 28.3333) along direction (0, -1, 0) blind 16 on bodies 1 bodies 1
extrude "Extrude61" add 1 faces at (-70.3333, 78, -46) along direction (0, -1, 0) blind 16 on bodies 1 bodies 1
extrude "Extrude62" cut 1 faces at (-70.5333, 83, 26.6667) along direction (0, -1, 0) blind 16 on bodies 1 bodies 1
extrude "Extrude63" cut 1 faces at (-64.3333, 78, -19) along direction (0, -1, 0) blind 16 on bodies 1 bodies 1
extrude "Extrude64" cut 1 faces at (-70.5333, 83, -42.6667) along direction (0, -1, 0) blind 16 on bodies 1 bodies 1
extrude "Extrude65" cut 1 faces at (-68.8, 96.3333, 26.6667) along direction (1, 0, 0) blind 0.8 on bodies 1 bodies 1
extrude "Extrude66" cut 1 faces at (-68.8, 96.3333, -44.3333) along direction (1, 0, 0) blind 0.8 on bodies 1 bodies 1
extrude "Extrude67" cut 1 faces at (-216.3333, 125.1667, 38.2) along direction (0, 0, -1) blind 0.9 on bodies 1 bodies 1
extrude "Extrude68" cut 1 faces at (-98.6667, 95.3333, 38.2) along direction (0, 0, -1) blind 0.9 on bodies 1 bodies 1
sketch "Sketch30" plane through (0, 155, 0) normal (0, 1, 0) x (-1, 0, 0)
  line L0 (97, 37.3) -> (97, 51.2)
  line L1 (97, 51.2) -> (218, 51.2)
  line L2 (218, 51.2) -> (218, 37.3)
  line L3 (218, 37.3) -> (213, 37.3)
  line L4 (213, 37.3) -> (213, 32.3)
  line L5 (213, 32.3) -> (223, 32.3)
  line L6 (223, 32.3) -> (223, 51.2)
  line L7 (223, 51.2) -> (249, 51.2)
  line L8 (249, 51.2) -> (249, 35)
  line L9 (249, 35) -> (236, 35)
  line L10 (236, 35) -> (236, 25)
  line L11 (236, 25) -> (241, 25)
  line L12 (241, 25) -> (241, 30)
  line L13 (241, 30) -> (247, 30)
  line L14 (247, 30) -> (247, 25)
  line L15 (247, 25) -> (254, 25)
  line L16 (254, 25) -> (254, -41)
  line L17 (254, -41) -> (247, -41)
  line L18 (247, -41) -> (247, -46)
  line L19 (247, -46) -> (241, -46)
  line L20 (241, -46) -> (241, -41)
  line L21 (241, -41) -> (236, -41)
  line L22 (236, -41) -> (236, -56)
  line L23 (236, -56) -> (249, -56)
  line L24 (249, -56) -> (249, -66)
  line L25 (249, -66) -> (259, -66)
  line L26 (259, -66) -> (259, 56.2)
  line L27 (259, 56.2) -> (56, 56.2)
  line L28 (56, 56.2) -> (56, -66)
  line L29 (56, -66) -> (66, -66)
  line L30 (66, -66) -> (66, -56)
  line L31 (66, -56) -> (79, -56)
  line L32 (79, -56) -> (79, -41)
  line L33 (79, -41) -> (74, -41)
  line L34 (74, -41) -> (74, -46)
  line L35 (74, -46) -> (68, -46)
  line L36 (68, -46) -> (68, -41)
  line L37 (68, -41) -> (61, -41)
  line L38 (61, -41) -> (61, 25)
  line L39 (61, 25) -> (68, 25)
  line L40 (68, 25) -> (68, 30)
  line L41 (68, 30) -> (74, 30)
  line L42 (74, 30) -> (74, 25)
  line L43 (74, 25) -> (79, 25)
  line L44 (79, 25) -> (79, 35)
  line L45 (79, 35) -> (66, 35)
  line L46 (66, 35) -> (66, 51.2)
  line L47 (66, 51.2) -> (92, 51.2)
  line L48 (92, 51.2) -> (92, 32.3)
  line L49 (92, 32.3) -> (102, 32.3)
  line L50 (102, 32.3) -> (102, 37.3)
  line L51 (102, 37.3) -> (97, 37.3)
  line L52 (61, 56.2) -> (56, 56.2)
  line L53 (56, 56.2) -> (56, -66)
  line L54 (56, -66) -> (61, -66)
  line L55 (61, -66) -> (61, 56.2)
  line L56 (254, 56.2) -> (259, 56.2)
  line L57 (259, 56.2) -> (259, -66)
  line L58 (259, -66) -> (254, -66)
  line L59 (254, -66) -> (254, 56.2)
  line L60 (61, 56.2) -> (254, 56.2)
  line L61 (254, 56.2) -> (254, 51.2)
  line L62 (254, 51.2) -> (61, 51.2)
  line L63 (61, 51.2) -> (61, 56.2)
  constraint horizontal L52
  constraint vertical L53
  constraint horizontal L54
  constraint vertical L55
  constraint coincident L28.end L29.start
  constraint coincident L27 L52.start
  constraint horizontal L56
  constraint vertical L57
  constraint horizontal L58
  constraint vertical L59
  constraint coincident L25.end L26.start
  constraint coincident L27 L56.start
  constraint horizontal L60
  constraint vertical L61
  constraint horizontal L62
  constraint vertical L63
  constraint coincident L59 L61.end
extrude "Extrude69" add sketch "Sketch30" along normal blind 5 contours L1 L7 L27 L47 L55 L59 L60 L61 L62 L63 | L27 L28 L29 L38 L52 L53 L54 L55 L63 | L16 L25 L26 L27 L56 L57 L58 L59 L61 bodies 1
extrude "Extrude70" cut 1 faces at (-176, 62.1667, 38.2) along direction (0, 0, 1) blind 7 on bodies 1 bodies 1
extrude "Extrude71" add 1 faces at (-74.6667, 93, -56) along direction (0, 0, -1) blind 10 on bodies 1 bodies 1
extrude "Extrude72" add 1 faces at (-244.6667, 93, -56) along direction (0, 0, -1) blind 10 on bodies 1 bodies 1
extrude "Extrude73" cut 1 faces at (-70, 96.3333, -46) along direction (0, 0, -1) blind 10 on bodies 1 bodies 1
extrude "Extrude74" cut 1 faces at (-63.3333, 94.6667, -41) along direction (0, 0, -1) blind 10 on bodies 1 bodies 1
extrude "Extrude75" add 1 faces at (-63.3333, 94.6667, 25) along direction (0, 0, -1) blind 10 on bodies 1 bodies 1
extrude "Extrude76" add 1 faces at (-70, 125.6667, 30) along direction (0, 0, -1) blind 10 on bodies 1 bodies 1
extrude "Extrude77" cut 1 faces at (-70, 96.3333, -56) along direction (0, 0, -1) blind 5 on bodies 1 bodies 1
extrude "Extrude78" cut 1 faces at (-63.3333, 94.6667, -51) along direction (0, 0, -1) blind 5 on bodies 1 bodies 1
extrude "Extrude79" add 1 faces at (-63.3333, 94.6667, 15) along direction (0, 0, -1) blind 5 on bodies 1 bodies 1
extrude "Extrude80" add 1 faces at (-70, 125.6667, 20) along direction (0, 0, -1) blind 5 on bodies 1 bodies 1
extrude "Extrude81" cut 1 faces at (-70.3333, 124, 35) along direction (0, 0, -1) blind 15 on bodies 1 bodies 1
extrude "Extrude82" cut 1 faces at (-243, 128.3333, -46) along direction (0, 0, -1) blind 15 on bodies 1 bodies 1
extrude "Extrude83" cut 1 faces at (-242, 66.3333, -41) along direction (0, 0, -1) blind 15 on bodies 1 bodies 1
extrude "Extrude84" add 1 faces at (-251.6667, 94.6667, 25) along direction (0, 0, -1) blind 15 on bodies 1 bodies 1
extrude "Extrude85" add 1 faces at (-245, 96.3333, 30) along direction (0, 0, -1) blind 15 on bodies 1 bodies 1
extrude "Extrude86" cut 1 faces at (-244.6667, 93, 35) along direction (0, 0, -1) blind 15 on bodies 1 bodies 1
extrude "Extrude87" cut 1 faces at (-98.6667, 92, 32.3) along direction (0, 0, 1) blind 5 on bodies 1 bodies 1
sketch "Sketch31" plane through (0, 0, 37.3) normal (0, 0, -1) x (-1, 0, 0)
  line L0 (97, 65.5) -> (97, 155)
  line L1 (97, 155) -> (92, 155)
  line L2 (92, 155) -> (92, 60.5)
  line L3 (92, 60.5) -> (102, 60.5)
  line L4 (102, 60.5) -> (102, 65.5)
  line L5 (102, 65.5) -> (97, 65.5)
  line L6 (102, 60.5) -> (92, 60.5)
  line L7 (92, 60.5) -> (92, 155)
  line L8 (92, 155) -> (102, 155)
  line L9 (102, 155) -> (102, 60.5)
  constraint horizontal L6
  constraint vertical L7
  constraint horizontal L8
  constraint vertical L9
  constraint coincident L1.end L2.start
  constraint coincident L3.end L4.start
extrude "Extrude88" add sketch "Sketch31" against normal blind 5 contours L0 L5 L8 L9 bodies 1
extrude "Extrude89" cut 1 faces at (-219.6667, 92, 32.3) along direction (0, 0, 1) blind 5 on bodies 1 bodies 1
sketch "Sketch32" plane through (0, 0, 37.3) normal (0, 0, -1) x (-1, 0, 0)
  line L0 (218, 65.5) -> (213, 65.5)
  line L1 (213, 65.5) -> (213, 60.5)
  line L2 (213, 60.5) -> (223, 60.5)
  line L3 (223, 60.5) -> (223, 155)
  line L4 (223, 155) -> (218, 155)
  line L5 (218, 155) -> (218, 65.5)
  line L6 (213, 60.5) -> (223, 60.5)
  line L7 (223, 60.5) -> (223, 155)
  line L8 (223, 155) -> (213, 155)
  line L9 (213, 155) -> (213, 60.5)
  constraint horizontal L6
  constraint vertical L7
  constraint horizontal L8
  constraint vertical L9
  constraint coincident L3.end L4.start
  constraint coincident L1.end L2.start
extrude "Extrude90" add sketch "Sketch32" against normal blind 5 contours L0 L5 L8 L9 bodies 1
sketch "Sketch33" plane through (0, 155, 0) normal (0, 1, 0) x (-1, 0, 0)
  line L0 (213, 37.3) -> (223, 37.3)
  line L1 (223, 37.3) -> (223, 51.2)
  line L2 (223, 51.2) -> (218, 51.2)
  line L3 (218, 51.2) -> (218, 42.3)
  line L4 (218, 42.3) -> (213, 42.3)
  line L5 (213, 42.3) -> (213, 37.3)
  line L6 (223, 51.2) -> (249, 51.2)
  line L7 (249, 51.2) -> (249, 20)
  line L8 (249, 20) -> (223, 20)
  line L9 (223, 20) -> (223, 51.2)
  point P0 (249, 20)
  constraint horizontal L6
  constraint vertical L7
  constraint horizontal L8
  constraint vertical L9
  constraint coincident P0 L7.end
  constraint coincident L1.end L2.start
extrude "Extrude91" add sketch "Sketch33" against normal blind 5 contours L1 L6 L7 L8 L9 bodies 1